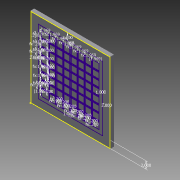
# Autodesk Inventor part: chess-board
Saved by Autodesk Inventor 2015 (Build 190159000, 159)
## iProperties
Created: 2014-12-29
Part Number: chess-board
Material: Generic
Document SubType Name: Modeling
Designer: TechShop Member
Density: 1 g/cm^3
Appearance: Default
Author: TechShop Member
Autodesk Inventor part; units mm, degrees
ref_plane "YZ Plane" through (0, 0, 0) normal (1, 0, 0) x (0, 1, 0)
ref_plane "XZ Plane" through (0, 0, 0) normal (0, 1, 0) x (-1, 0, 0)
ref_plane "XY Plane" through (0, 0, 0) normal (0, 0, 1) x (1, 0, 0)
sketch "Sketch1" plane through (0, 0, 0) normal (0, 0, 1) x (1, 0, 0)
  line L0 (0, 0) -> (558.8, 0)
  line L1 (558.8, 0) -> (558.8, 558.8)
  line L2 (558.8, 558.8) -> (0, 558.8)
  line L3 (0, 558.8) -> (0, 0)
  dimension "d0" = 558.8
  dimension "d1" = 558.8
  constraints: 8 end point, 2 parallel, 1 horizontal, 1 perpendicular
  measures "d0" distance of L1.end L2.end
  measures "d1" distance of L0.end L1.end
extrude "Extrusion1" add sketch "Sketch1" along normal blind 25.4
fillet "Fillet1" radius 3.175 1 edges at (279.4, 558.8, 25.4)
fillet "Fillet2" radius 3.175 3 edges at (0, 557.8701, 24.4701) (0, 558.8, 11.1125) (0, 277.8125, 25.4)
fillet "Fillet3" radius 3.175 3 edges at (558.8, 557.8701, 24.4701) (558.8, 558.8, 11.1125) (558.8, 277.8125, 25.4)
fillet "Fillet4" radius 3.175 5 edges at (557.8701, 0, 24.4701) (558.8, 0, 11.1125) (0.9299, 0, 24.4701) (0, 0, 11.1125) (279.4, 0, 25.4)
sketch "Sketch2" plane through (0, 0, 25.4) normal (0, 0, 1) x (1, 0, 0)
  line L0 (555.625, 3.175) -> (3.175, 3.175) projected
  line L1 (555.625, 555.625) -> (555.625, 3.175) projected
  line L2 (3.175, 555.625) -> (555.625, 555.625) projected
  line L3 (3.175, 3.175) -> (3.175, 555.625) projected
  line L4 (79.375, 79.375) -> (79.375, 479.425)
  line L5 (79.375, 479.425) -> (479.425, 479.425)
  line L6 (479.425, 479.425) -> (479.425, 79.375)
  line L7 (479.425, 79.375) -> (79.375, 79.375)
  line L8 (129.3812, 479.425) -> (129.3812, 79.375)
  line L9 (429.4187, 479.425) -> (429.4187, 79.375)
  line L10 (379.4125, 479.425) -> (379.4125, 79.375)
  line L11 (179.3875, 479.425) -> (179.3875, 79.375)
  line L12 (229.3937, 479.425) -> (229.3937, 79.375)
  line L13 (329.4062, 479.425) -> (329.4062, 79.375)
  line L14 (279.4, 479.425) -> (279.4, 79.375)
  line L15 (79.375, 129.3813) -> (479.425, 129.3813)
  line L16 (79.375, 179.3875) -> (479.425, 179.3875)
  line L17 (79.375, 429.4188) -> (479.425, 429.4188)
  line L18 (79.375, 379.4125) -> (479.425, 379.4125)
  line L19 (79.375, 329.4063) -> (479.425, 329.4063)
  line L20 (79.375, 279.4) -> (479.425, 279.4)
  line L21 (79.375, 229.3938) -> (479.425, 229.3938)
  line L22 (53.975, 504.825) -> (504.825, 504.825)
  line L23 (504.825, 504.825) -> (504.825, 53.975)
  line L24 (504.825, 53.975) -> (53.975, 53.975)
  line L25 (53.975, 53.975) -> (53.975, 504.825)
  line L26 (134.4612, 479.425) -> (134.4612, 79.375)
  line L27 (129.3812, 479.425) -> (129.3812, 79.375)
  line L28 (174.3075, 479.425) -> (174.3075, 79.375)
  line L29 (184.4675, 479.425) -> (184.4675, 79.375)
  line L30 (224.3137, 479.425) -> (224.3137, 79.375)
  line L31 (234.4737, 479.425) -> (234.4737, 79.375)
  line L32 (274.32, 479.425) -> (274.32, 79.375)
  line L33 (284.48, 479.425) -> (284.48, 79.375)
  line L34 (324.3262, 479.425) -> (324.3262, 79.375)
  line L35 (334.4862, 479.425) -> (334.4862, 79.375)
  line L36 (374.3325, 479.425) -> (374.3325, 79.375)
  line L37 (384.4925, 479.425) -> (384.4925, 79.375)
  line L38 (424.3387, 479.425) -> (424.3387, 79.375)
  line L39 (434.4987, 479.425) -> (434.4987, 79.375)
  line L40 (479.425, 124.3013) -> (79.375, 124.3013)
  line L41 (79.375, 134.4613) -> (479.425, 134.4613)
  line L42 (479.425, 174.3075) -> (79.375, 174.3075)
  line L43 (79.375, 184.4675) -> (479.425, 184.4675)
  line L44 (479.425, 224.3138) -> (79.375, 224.3138)
  line L45 (79.375, 234.4737) -> (479.425, 234.4738)
  line L46 (479.425, 274.32) -> (79.375, 274.32)
  line L47 (79.375, 284.48) -> (479.425, 284.48)
  line L48 (479.425, 324.3263) -> (79.375, 324.3263)
  line L49 (479.425, 334.4863) -> (79.375, 334.4863)
  line L50 (79.375, 374.3325) -> (479.425, 374.3325)
  line L51 (479.425, 384.4925) -> (79.375, 384.4925)
  line L52 (79.375, 424.3388) -> (479.425, 424.3388)
  line L53 (479.425, 434.4988) -> (79.375, 434.4988)
  point P0 (0, 0)
  dimension "d12" = 50.0063
  dimension "d13" = 50.0063
  dimension "d14" = 50.0063
  dimension "d15" = 50.0063
  dimension "d16" = 50.0063
  dimension "d17" = 50.0063
  dimension "d18" = 50.0063
  dimension "d19" = 50.0063
  dimension "d20" = 50.0063
  dimension "d21" = 50.0063
  dimension "d22" = 50.0063
  dimension "d23" = 50.0063
  dimension "d24" = 50.0063
  dimension "d25" = 50.0063
  dimension "d26" = 50.0063
  dimension "d27" = 50.0063
  dimension "d28" = 25.4
  dimension "d29" = 25.4
  dimension "d30" = 25.4
  dimension "d31" = 25.4
  dimension "d32" = 50.8
  dimension "d33" = 50.8
  dimension "d34" = 50.8
  dimension "d35" = 50.8
  dimension "d36" = 5.08
  dimension "d37" = 5.08
  dimension "d38" = 5.08
  dimension "d39" = 5.08
  dimension "d40" = 5.08
  dimension "d41" = 5.08
  dimension "d42" = 5.08
  dimension "d43" = 5.08
  dimension "d44" = 5.08
  dimension "d45" = 5.08
  dimension "d46" = 5.08
  dimension "d47" = 5.08
  dimension "d48" = 5.08
  dimension "d49" = 5.08
  dimension "d50" = 5.08
  dimension "d51" = 5.08
  dimension "d52" = 5.08
  dimension "d53" = 5.08
  dimension "d54" = 5.08
  dimension "d55" = 5.08
  dimension "d56" = 5.08
  dimension "d57" = 5.08
  dimension "d58" = 5.08
  dimension "d59" = 5.08
  dimension "d60" = 5.08
  dimension "d61" = 5.08
  dimension "d62" = 5.08
  constraints: 92 end point, 24 vertical, 22 horizontal, 2 parallel, 1 perpendicular, 95 other
  measures "d13" distance between parallel lines of L8 L11
  measures "d14" distance between parallel lines of L12 L11
  measures "d15" distance between parallel lines of L14 L12
  measures "d16" distance between parallel lines of L13 L14
  measures "d17" distance between parallel lines of L10 L13
  measures "d18" distance between parallel lines of L9 L10
  measures "d21" distance between parallel lines of L18 L17
  measures "d22" distance between parallel lines of L19 L18
  measures "d23" distance between parallel lines of L20 L19
  measures "d24" distance between parallel lines of L21 L20
  measures "d25" distance between parallel lines of L16 L21
  measures "d26" distance between parallel lines of L15 L16
  measures "d32" distance between parallel lines of L22 L2
  measures "d33" distance between parallel lines of L0 L24
  measures "d34" distance between parallel lines of L1 L23
  measures "d35" distance between parallel lines of L25 L3
  measures "d36" distance between parallel lines of L17 L53
  measures "d37" distance between parallel lines of L8 L26
  measures "d38" distance between parallel lines of L17 L52
  measures "d39" distance between parallel lines of L18 L51
  measures "d40" distance between parallel lines of L18 L50
  measures "d41" distance between parallel lines of L19 L49
  measures "d42" distance between parallel lines of L48 L19
  measures "d43" distance between parallel lines of L20 L47
  measures "d44" distance between parallel lines of L46 L20
  measures "d45" distance between parallel lines of L21 L45
  measures "d46" distance between parallel lines of L44 L21
  measures "d47" distance between parallel lines of L16 L43
  measures "d48" distance between parallel lines of L16 L42
  measures "d49" distance between parallel lines of L15 L41
  measures "d50" distance between parallel lines of L15 L40
  measures "d51" distance between parallel lines of L11 L28
  measures "d52" distance between parallel lines of L11 L29
  measures "d53" distance between parallel lines of L12 L30
  measures "d54" distance between parallel lines of L12 L31
  measures "d55" distance between parallel lines of L14 L32
  measures "d56" distance between parallel lines of L14 L33
  measures "d57" distance between parallel lines of L13 L34
  measures "d58" distance between parallel lines of L13 L35
  measures "d59" distance between parallel lines of L10 L36
  measures "d60" distance between parallel lines of L10 L37
  measures "d61" distance between parallel lines of L9 L38
  measures "d62" distance between parallel lines of L9 L39
equation "\"d13\" = d12"
equation "\"d14\" = d12"
equation "\"d15\" = d12"
equation "\"d16\" = d12"
equation "\"d17\" = d12"
equation "\"d18\" = d12"
equation "\"d20\" = d12"
equation "\"d21\" = d12"
equation "\"d22\" = d12"
equation "\"d23\" = d12"
equation "\"d24\" = d12"
equation "\"d25\" = d12"
equation "\"d26\" = d12"
equation "\"d37\" = d36"
equation "\"d38\" = d36"
equation "\"d39\" = d36"
equation "\"d40\" = d39"
equation "\"d41\" = d39"
equation "\"d42\" = d41"
equation "\"d43\" = d41"
equation "\"d44\" = d41"
equation "\"d45\" = d43"
equation "\"d46\" = d45"
equation "\"d47\" = d45"
equation "\"d48\" = d47"
equation "\"d49\" = d48"
equation "\"d50\" = d49"
equation "\"d51\" = d49"
equation "\"d52\" = d49"
equation "\"d53\" = d52"
equation "\"d54\" = d51"
equation "\"d55\" = d53"
equation "\"d56\" = d55"
equation "\"d57\" = d55"
equation "\"d58\" = d56"
equation "\"d59\" = d57"
equation "\"d60\" = d57"
equation "\"d61\" = d60"
equation "\"d62\" = d59"
body "Solid1"
